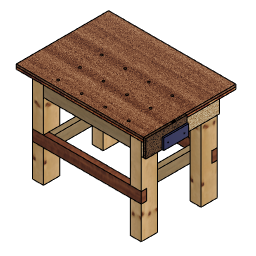
workbench (Autodesk Fusion 360 design; units mm, degrees)
Autodesk Fusion 360 part; units mm, degrees
note: some values were not read from the file. Set by a fixed rule: which face or edge a step refers to.
sketch "Sketch1" plane through (0, 0, 0) normal (0, 0, 1) x (1, 0, 0)
  line L0 (0, 0) -> (100, 0)
  line L1 (100, 0) -> (100, 150)
  line L2 (100, 150) -> (0, 150)
  line L3 (0, 150) -> (0, 0)
  dimension "d1" = 100
  dimension "d2" = 150
  constraint horizontal L0
  constraint vertical L1
  constraint horizontal L2
  constraint vertical L3
  constraint coincident L0.start L3.end
  measures "d1" distance of L0.start L0.end
  measures "d2" distance of L0.start L2.end
extrude "Extrude1" add sketch "Sketch1" along normal blind 800 makes body 1
sketch "Sketch2" plane through (0, 0, 0) normal (-1, 0, 0) x (0, -1, 0)
  line L0 (-150, 0) -> (0, 0)
  line L1 (0, 0) -> (0, 800)
  line L2 (0, 800) -> (-150, 800)
  line L3 (-150, 800) -> (-150, 0)
  line L4 (0, 300) -> (-50, 300)
  line L5 (-50, 300) -> (-50, 400)
  line L6 (-50, 400) -> (0, 400)
  line L7 (0, 400) -> (0, 300)
  dimension "d5" = 50
  dimension "d6" = 100
  constraint horizontal L4
  constraint vertical L5
  constraint horizontal L6
  constraint vertical L7
  constraint coincident L1 L4.start
  measures "d5" distance of L4.start L4.end
  measures "d6" distance of L4.end L5.end
extrude "Extrude2" cut sketch "Sketch2" against normal blind 100 contours L1 L4 L5 L6 L7 bodies 1
sketch "Sketch4" plane through (0, 150, 0) normal (0, -1, 0) x (1, 0, 0)
  line L0 (0, 400) -> (100, 400)
  line L1 (100, 400) -> (100, 800)
  line L2 (100, 800) -> (0, 800)
  line L3 (0, 800) -> (0, 400)
  line L4 (0, 800) -> (150, 800)
  line L5 (150, 800) -> (150, 700)
  line L6 (150, 700) -> (0, 700)
  line L7 (0, 700) -> (0, 800)
  line L8 (100, 0) -> (0, 0)
  line L9 (0, 0) -> (0, 800)
  line L10 (0, 800) -> (100, 800)
  line L11 (100, 800) -> (100, 0)
  dimension "d15" = 100
  dimension "d16" = 150
  constraint horizontal L4
  constraint vertical L5
  constraint horizontal L6
  constraint vertical L7
  constraint coincident L2.end L3.start
  measures "d15" distance of L2.end L6.end
  measures "d16" distance of L2.end L4.end
extrude "Extrude5" cut sketch "Sketch4" along normal blind 100 contours L1 L2 L3 L4 L6 L7 L9 L10 L11 | L1 L4 L5 L6 L11 bodies 1
extrude "Extrude6" add sketch "Sketch2" against normal blind 1000 separate body contours L1 L4 L5 L6 L7 makes body 2
extrude "Extrude7" add sketch "Sketch4" against normal blind 500 separate body contours L1 L2 L3 L4 L6 L7 L9 L10 L11 | L1 L4 L5 L6 L11 makes body 3
extrude "Extrude10" add 1 faces at (33.3333, 150, 766.6667) along direction (0, -1, 0) blind 100 on bodies 3 bodies 3
mirror "Mirror1" about plane through (0, 0, 0) normal (1, 0, 0) of bodies 1 makes body 4
move_body "Move3" bodies 4 to x (1, 0, 0) y (0, 1, 0) z (0, 0, 1) at (1000, 0, 0)
copy_body "CopyPasteBodies3" bodies 3 makes body 5
move_body "Move4" bodies 5 to x (1, 0, 0) y (0, 1, 0) z (0, 0, 1) at (850, 0, 0)
mirror "Mirror2" about plane through (0, 0, 0) normal (0, 1, 0) of bodies 1 makes body 6
move_body "Move5" bodies 6 to x (1, 0, 0) y (0, 1, 0) z (0, 0, 1) at (0, 700, 0)
copy_body "CopyPasteBodies4" bodies 2 makes body 7
move_body "Move6" bodies 7 to x (1, 0, 0) y (0, 1, 0) z (0, 0, 1) at (0, 650, 0)
mirror "Mirror3" about plane through (0, 0, 0) normal (1, 0, 0) of bodies 6 makes body 8
move_body "Move7" bodies 8 to x (1, 0, 0) y (0, 1, 0) z (0, 0, 1) at (1000, 0, 0)
sketch "Sketch5" plane through (0, 650, 0) normal (0, -1, 0) x (1, 0, 0)
  line L0 (0, 400) -> (0, 300)
  line L1 (0, 300) -> (1000, 300)
  line L2 (1000, 300) -> (1000, 400)
  line L3 (1000, 400) -> (0, 400)
  line L4 (100, 400) -> (150, 400)
  line L5 (150, 400) -> (150, 300)
  line L6 (150, 300) -> (100, 300)
  line L7 (100, 300) -> (100, 400)
  constraint horizontal L4
  constraint vertical L5
  constraint horizontal L6
  constraint vertical L7
  constraint coincident L1 L5.end
  constraint coincident L3 L4.start
extrude "Extrude8" add sketch "Sketch5" along normal blind 600 separate body contours L1 L3 L4 L5 L6 L7 makes body 9
copy_body "CopyPasteBodies5" bodies 9 makes body 10
move_body "Move8" bodies 10 to x (1, 0, 0) y (0, 1, 0) z (0, 0, 1) at (750, 0, 0)
sketch "Sketch7" plane through (100, 0, 0) normal (1, 0, 0) x (0, 1, 0)
  line L0 (50, 700) -> (50, 800)
  line L1 (50, 800) -> (0, 800)
  line L2 (0, 800) -> (0, 400)
  line L3 (0, 400) -> (50, 400)
  line L4 (50, 400) -> (50, 300)
  line L5 (50, 300) -> (0, 300)
  line L6 (0, 300) -> (0, 0)
  line L7 (0, 0) -> (150, 0)
  line L8 (150, 0) -> (150, 700)
  line L9 (150, 700) -> (50, 700)
  line L10 (0, 800) -> (50, 800)
  line L11 (50, 800) -> (50, 700)
  line L12 (50, 700) -> (0, 700)
  line L13 (0, 700) -> (0, 800)
  constraint horizontal L10
  constraint vertical L11
  constraint horizontal L12
  constraint vertical L13
  constraint coincident L0.start L9.end
  constraint coincident L1.end L2.start
extrude "Extrude11" add sketch "Sketch7" along normal blind 800 separate body contours L0 L1 L2 L10 L11 L12 L13 makes body 11
copy_body "CopyPasteBodies6" bodies 11 makes body 12
move_body "Move9" bodies 12 to x (1, 0, 0) y (0, 1, 0) z (0, 0, 1) at (0, 650, 0)
sketch "Sketch8" plane through (0, 0, 800) normal (0, 0, 1) x (-1, 0, 0)
  line L0 (-1000, -50) -> (-900, -50)
  line L1 (-900, -50) -> (-900, 0)
  line L2 (-900, 0) -> (-1000, 0)
  line L3 (-1000, 0) -> (-1000, -50)
  line L4 (-1000, 0) -> (150, 0)
  line L5 (150, 0) -> (150, -850)
  line L6 (150, -850) -> (-1000, -850)
  line L7 (-1000, -850) -> (-1000, 0)
  constraint horizontal L4
  constraint vertical L5
  constraint horizontal L6
  constraint vertical L7
  constraint coincident L2.end L3.start
extrude "Extrude12" add sketch "Sketch8" along normal blind 21 separate body makes body 13
copy_body "CopyPasteBodies7" bodies 13 makes body 14
move_body "Move10" bodies 14 to x (1, 0, 0) y (0, 1, 0) z (0, 0, 1) at (0, 0, 21)
sketch "Sketch9" plane through (1000, 0, 0) normal (1, 0, 0) x (0, 1, 0)
  line L0 (50, 700) -> (650, 700)
  line L1 (650, 700) -> (650, 800)
  line L2 (650, 800) -> (50, 800)
  line L3 (50, 800) -> (50, 700)
  line L4 (150, 700) -> (380, 700)
  line L5 (380, 700) -> (380, 780)
  line L6 (380, 780) -> (150, 780)
  line L7 (150, 780) -> (150, 700)
  dimension "d39" = 230
  dimension "d40" = 80
  constraint horizontal L4
  constraint vertical L5
  constraint horizontal L6
  constraint vertical L7
  constraint coincident L0 L4.start
  measures "d39" distance of L5.end L6.end
  measures "d40" distance of L4.start L6.end
extrude "Extrude14" cut sketch "Sketch9" against normal blind 15 contours L0 L4 L5 L6 L7 bodies 5
extrude "Extrude15" add 1 faces at (985, 226.6667, 753.3333) along direction (1, 0, 0) blind 15 separate body on bodies 5 makes body 15
extrude "Extrude16" add 1 faces at (990, 226.6667, 700) along direction (0, 0, -1) blind 20 on bodies 15 bodies 15
sketch "Sketch10" plane through (985, 0, 0) normal (-1, 0, 0) x (0, -1, 0)
  line L0 (-150, 680) -> (-150, 780)
  line L1 (-150, 780) -> (-380, 780)
  line L2 (-380, 780) -> (-380, 680)
  line L3 (-380, 680) -> (-150, 680)
  line L4 (-380, 680) -> (-150, 680)
  line L5 (-150, 680) -> (-150, 700)
  line L6 (-150, 700) -> (-380, 700)
  line L7 (-380, 700) -> (-380, 680)
  constraint horizontal L4
  constraint vertical L5
  constraint horizontal L6
  constraint vertical L7
  constraint coincident L0 L5.end
  constraint coincident L2.end L3.start
extrude "Extrude17" add sketch "Sketch10" along normal blind 120 contours L0 L2 L3 L4 L5 L6 L7 bodies 15
sketch "Sketch11" plane through (0, 0, 700) normal (0, 0, 1) x (-1, 0, 0)
  line L0 (-985, -150) -> (-985, -380)
  line L1 (-985, -380) -> (-865, -380)
  line L2 (-865, -380) -> (-865, -150)
  line L3 (-865, -150) -> (-985, -150)
  line L4 (-865, -150) -> (-985, -150)
  line L5 (-985, -150) -> (-985, -158.5)
  line L6 (-985, -158.5) -> (-865, -158.5)
  line L7 (-865, -158.5) -> (-865, -150)
  dimension "d49" = 8.5
  constraint horizontal L4
  constraint vertical L5
  constraint horizontal L6
  constraint vertical L7
  constraint coincident L0 L5.end
  constraint coincident L2.end L3.start
  measures "d49" distance of L2.end L6.end
extrude "Extrude18" cut sketch "Sketch11" against normal blind 20 contours L0 L2 L3 L4 L5 L6 L7 bodies 15
sketch "Sketch12" plane through (0, 0, 700) normal (0, 0, 1) x (-1, 0, 0)
  line L0 (-865, -158.5) -> (-985, -158.5)
  line L1 (-985, -158.5) -> (-985, -380)
  line L2 (-985, -380) -> (-865, -380)
  line L3 (-865, -380) -> (-865, -158.5)
  line L4 (-865, -380) -> (-985, -380)
  line L5 (-985, -380) -> (-985, -371.5)
  line L6 (-985, -371.5) -> (-865, -371.5)
  line L7 (-865, -371.5) -> (-865, -380)
  dimension "d52" = 8.5
  constraint horizontal L4
  constraint vertical L5
  constraint horizontal L6
  constraint vertical L7
  constraint coincident L1 L5.end
  constraint coincident L2.end L3.start
  measures "d52" distance of L2.end L6.end
extrude "Extrude19" cut sketch "Sketch12" against normal blind 20 contours L1 L2 L3 L4 L5 L6 L7 bodies 15
sketch "Sketch13" plane through (0, 0, 700) normal (0, 0, 1) x (-1, 0, 0)
  line L0 (-985, -371.5) -> (-865, -371.5)
  line L1 (-865, -371.5) -> (-865, -158.5)
  line L2 (-865, -158.5) -> (-985, -158.5)
  line L3 (-985, -158.5) -> (-985, -371.5)
  circle A0 centre (-962.5, -176) radius 7.5
  circle A1 centre (-962.5, -354) radius 7.5
  circle A2 centre (-885.5, -184) radius 7.5
  circle A3 centre (-885.5, -346) radius 7.5
  dimension "d55" = 15
  dimension "d56" = 17.5
  dimension "d57" = 22.5
  dimension "d58" = 15
  dimension "d59" = 17.5
  dimension "d60" = 22.5
  dimension "d61" = 15
  dimension "d62" = 15
  dimension "d63" = 99.5
  dimension "d64" = 99.5
  dimension "d65" = 25.5
  dimension "d66" = 25.5
  measures "d55" diameter of A0
  measures "d56" distance of L2 A0.centre
  measures "d57" distance of L3 A0.centre
  measures "d58" diameter of A1
  measures "d59" distance of L0 A1.centre
  measures "d60" distance of L3 A1.centre
  measures "d61" diameter of A2
  measures "d62" diameter of A3
  measures "d63" distance of L3 A2.centre
  measures "d64" distance of L3 A3.centre
  measures "d65" distance of L2 A2.centre
  measures "d66" distance of L0 A3.centre
extrude "Extrude20" cut sketch "Sketch13" against normal blind 20 contours A0 | A1 | A2 | A3 bodies 15
sketch "Sketch14" plane through (985, 0, 0) normal (-1, 0, 0) x (0, -1, 0)
  line L0 (-371.5, 700) -> (-158.5, 700)
  line L1 (-158.5, 700) -> (-158.5, 680)
  line L2 (-158.5, 680) -> (-150, 680)
  line L3 (-150, 680) -> (-150, 780)
  line L4 (-150, 780) -> (-380, 780)
  line L5 (-380, 780) -> (-380, 680)
  line L6 (-380, 680) -> (-371.5, 680)
  line L7 (-371.5, 680) -> (-371.5, 700)
  circle A0 centre (-340, 724) radius 4
  circle A1 centre (-190, 724) radius 4
  dimension "d69" = 8
  dimension "d70" = 8
  dimension "d71" = 40
  dimension "d72" = 40
  dimension "d73" = 56
  dimension "d74" = 56
  measures "d69" diameter of A0
  measures "d70" diameter of A1
  measures "d71" distance of L5 A0.centre
  measures "d72" distance of L3 A1.centre
  measures "d73" distance of L4 A0.centre
  measures "d74" distance of L4 A1.centre
extrude "Extrude21" cut sketch "Sketch14" against normal blind 15 contours A0 | A1 bodies 15
sketch "Sketch15" plane through (1000, 0, 0) normal (1, 0, 0) x (0, 1, 0)
  circle A0 centre (340, 724) radius 4
  circle A1 centre (190, 724) radius 4
  line L0 (150, 780) -> (150, 680)
  line L1 (150, 680) -> (380, 680)
  line L2 (380, 680) -> (380, 780)
  line L3 (380, 780) -> (150, 780)
  line L4 (380, 680) -> (0, 680)
  line L5 (0, 680) -> (0, 800)
  line L6 (0, 800) -> (380, 800)
  line L7 (380, 800) -> (380, 680)
  dimension "d77" = 380
  constraint horizontal L4
  constraint vertical L5
  constraint horizontal L6
  constraint vertical L7
  constraint coincident L1.end L2.start
  measures "d77" distance of L5.end L6.end
extrude "Extrude22" add sketch "Sketch15" along normal blind 21 separate body makes body 16
copy_body "CopyPasteBodies8" bodies 16 makes body 17
move_body "Move11" bodies 17 to x (1, 0, 0) y (0, 1, 0) z (0, 0, 1) at (21, 0, 0)
extrude "Extrude23" add 2 faces at (1007, 380, 713.3333) (1007, 380, 793.3333) along direction (0, 1, 0) blind 320 on bodies 16 bodies 16
extrude "Extrude24" add 2 faces at (1000, 16.6667, 807) (1000, 583.3333, 814) along direction (1, 0, 0) blind 21 on bodies 13 bodies 13
extrude "Extrude25" add 2 faces at (1000, 16.6667, 828) (1000, 583.3333, 835) along direction (1, 0, 0) blind 21 on bodies 14 bodies 14
extrude "Extrude26" add 1 faces at (1028, 126.6667, 800) along direction (0, 0, 1) blind 42 on bodies 17 bodies 17
sketch "Sketch17" plane through (0, 0, 842) normal (0, 0, 1) x (-1, 0, 0)
  line L0 (-1021, -850) -> (150, -850)
  line L1 (150, -850) -> (150, 0)
  line L2 (150, 0) -> (-1021, 0)
  line L3 (-1021, 0) -> (-1021, -850)
  circle A0 centre (-821, -265) radius 10
  circle A1 centre (-821, -65) radius 10
  circle A2 centre (-604.3333, -65) radius 10
  circle A3 centre (-604.3333, -265) radius 10
  circle A4 centre (-387.6667, -265) radius 10
  circle A5 centre (-387.6667, -65) radius 10
  circle A6 centre (-171, -65) radius 10
  circle A7 centre (-171, -265) radius 10
  line L4 (-821, -265) -> (-1058.3995, -265) construction
  line L5 (-1036.8104, -250) -> (-1026.8104, -250)
  line L6 (-1026.8104, -250) -> (-1026.8104, -280)
  line L7 (-1026.8104, -280) -> (-1036.8104, -280)
  line L8 (-1036.8104, -280) -> (-1036.8104, -250)
  line L9 (-1036.8104, -250) -> (-1026.8104, -280) construction
  line L10 (-1026.8104, -250) -> (-1036.8104, -280) construction
  line L11 (-985, -150) -> (-1000, -150)
  circle A8 centre (-821, -465) radius 10
  circle A9 centre (-604.3333, -465) radius 10
  circle A10 centre (-387.6667, -465) radius 10
  circle A11 centre (-171, -465) radius 10
  point P0 (-1031.8104, -265)
  dimension "d92" = 20
  dimension "d93" = 265
  dimension "d94" = 200
  dimension "d99" = 650
  dimension "d100" = -200
  dimension "d103" = 10
  dimension "d104" = 30
  dimension "d109" = 115
  constraint coincident A0.centre L4.start
  constraint horizontal L5
  constraint perpendicular L5 L6
  constraint parallel L5 L7
  constraint parallel L6 L8
  constraint coincident L9 P0
  constraint coincident L10 P0
  constraint coincident L4 P0
  constraint parallel L2 L4
  measures "d92" diameter of A0
  measures "d93" distance of L2 A0.centre
  measures "d94" distance of L3 A0.centre
  measures "d103" distance of L6.end L7.end
  measures "d104" distance of L5.end L6.end
  measures "d109" distance of P0 L11
extrude "Extrude28" cut sketch "Sketch17" against normal blind 42 contours A0 | A1 | A2 | A3 | A4 | A5 | A6 | A7 | L5 L6 L7 L8 | A8 | A9 | A10 | A11 bodies 17 14 13
sketch "Sketch16" plane through (1042, 0, 0) normal (1, 0, 0) x (0, 1, 0)
  circle A0 centre (190, 724) radius 4
  circle A1 centre (340, 724) radius 4
  line L0 (0, 842) -> (0, 680)
  line L1 (0, 680) -> (380, 680)
  line L2 (380, 680) -> (380, 842)
  line L3 (380, 842) -> (0, 842)
  line L4 (380, 680) -> (150, 680)
  line L5 (150, 680) -> (150, 780)
  line L6 (150, 780) -> (380, 780)
  line L7 (380, 780) -> (380, 680)
  dimension "d88" = 230
  dimension "d89" = 100
  constraint horizontal L4
  constraint vertical L5
  constraint horizontal L6
  constraint vertical L7
  constraint coincident L1.end L2.start
  measures "d88" distance of L5.end L6.end
  measures "d89" distance of L1.end L6.end
extrude "Extrude27" add sketch "Sketch16" along normal blind 15 separate body contours L1 L2 L4 L5 L6 L7 makes body 18
copy_body "Body->Comp1" bodies 1 removing the originals makes body 19 in component "ножка"
copy_body "Body->Comp2" bodies 2 removing the originals makes body 20 in component "перекладина длинная низ"
copy_body "Body->Comp3" bodies 7 removing the originals makes body 21 in component "перекладина длинная низ (1)"
copy_body "Body->Comp4" bodies 9 removing the originals makes body 22 in component "перекладина короткая низ"
copy_body "Body->Comp5" bodies 10 removing the originals makes body 23 in component "перекладина короткая низ (1)"
copy_body "Body->Comp6" bodies 3 removing the originals makes body 24 in component "перекладина короткая верх"
copy_body "Body->Comp7" bodies 4 removing the originals makes body 25 in component "ножка (1)"
copy_body "Body->Comp8" bodies 5 removing the originals makes body 26 in component "перекладина короткая верх (1)"
copy_body "Body->Comp9" bodies 6 removing the originals makes body 27 in component "ножка (2)"
copy_body "Body->Comp10" bodies 8 removing the originals makes body 28 in component "ножка (2) (1)"
copy_body "Body->Comp11" bodies 11 removing the originals makes body 29 in component "перекладина длинная верх"
copy_body "Body->Comp12" bodies 12 removing the originals makes body 30 in component "перекладина длинная верх (1)"
copy_body "Body->Comp13" bodies 13 removing the originals makes body 31 in component "столешница (фанера)"
copy_body "Body->Comp14" bodies 14 removing the originals makes body 32 in component "столешница (фанера)(1)"
copy_body "Body->Comp15" bodies 16 removing the originals makes body 33 in component "фанера"
copy_body "Body->Comp16" bodies 17 removing the originals makes body 34 in component "фанера (1)"
copy_body "Body->Comp17" bodies 15 removing the originals makes body 35 in component "тиски"
copy_body "Body->Comp18" bodies 18 removing the originals makes body 36 in component "тиски 2"
component "ножка" placed x (1, 0, 0) y (0, 1, 0) z (0, 0, 1) at (0, 0, 0)
component "перекладина длинная низ" placed x (1, 0, 0) y (0, 1, 0) z (0, 0, 1) at (0, 0, 0)
component "перекладина длинная низ (1)" placed x (1, 0, 0) y (0, 1, 0) z (0, 0, 1) at (0, 0, 0)
component "перекладина короткая низ" placed x (1, 0, 0) y (0, 1, 0) z (0, 0, 1) at (0, 0, 0)
component "перекладина короткая низ (1)" placed x (1, 0, 0) y (0, 1, 0) z (0, 0, 1) at (0, 0, 0)
component "перекладина короткая верх" placed x (1, 0, 0) y (0, 1, 0) z (0, 0, 1) at (0, 0, 0)
component "ножка (1)" placed x (1, 0, 0) y (0, 1, 0) z (0, 0, 1) at (0, 0, 0)
component "перекладина короткая верх (1)" placed x (1, 0, 0) y (0, 1, 0) z (0, 0, 1) at (0, 0, 0)
component "ножка (2)" placed x (1, 0, 0) y (0, 1, 0) z (0, 0, 1) at (0, 0, 0)
component "ножка (2) (1)" placed x (1, 0, 0) y (0, 1, 0) z (0, 0, 1) at (0, 0, 0)
component "перекладина длинная верх" placed x (1, 0, 0) y (0, 1, 0) z (0, 0, 1) at (0, 0, 0)
component "перекладина длинная верх (1)" placed x (1, 0, 0) y (0, 1, 0) z (0, 0, 1) at (0, 0, 0)
component "столешница (фанера)" placed x (1, 0, 0) y (0, 1, 0) z (0, 0, 1) at (0, 0, 0)
component "столешница (фанера)(1)" placed x (1, 0, 0) y (0, 1, 0) z (0, 0, 1) at (0, 0, 0)
component "фанера" placed x (1, 0, 0) y (0, 1, 0) z (0, 0, 1) at (0, 0, 0)
component "фанера (1)" placed x (1, 0, 0) y (0, 1, 0) z (0, 0, 1) at (0, 0, 0)
component "тиски" placed x (1, 0, 0) y (0, 1, 0) z (0, 0, 1) at (0, 0, 0)
component "тиски 2" placed x (1, 0, 0) y (0, 1, 0) z (0, 0, 1) at (0, 0, 0)
equation "d56 = 10 mm + ( 15 / 2 ) * 1 mm"
equation "d57 = 15 mm + ( 15 / 2 ) * 1 mm"
equation "d59 = 10 mm + ( 15 / 2 ) * 1 mm"
equation "d60 = 15 mm + ( 15 / 2 ) * 1 mm"
equation "d63 = 92 mm + ( 15 / 2 ) * 1 mm"
equation "d64 = 92 mm + ( 15 / 2 ) * 1 mm"
equation "d65 = 18 mm + ( 15 / 2 ) * 1 mm"
equation "d66 = 18 mm + ( 15 / 2 ) * 1 mm"
equation "d71 = 36 mm + 4 mm"
equation "d72 = 36 mm + 4 mm"
equation "d73 = 52 mm + 4 mm"
equation "d74 = 52 mm + 4 mm"
named bodies: "ножка", "перекладина длинная низ", "перекладина короткая верх", "ножка (1)", "перекладина короткая верх (1)", "ножка (2)", "перекладина длинная низ (1)", "ножка (2) (1)", "перекладина короткая низ", "перекладина короткая низ (1)", "перекладина длинная верх", "перекладина длинная верх (1)", "столешница (фанера)", "столешница", "столешница (фанера)(1)", "тиски", "фанера", "фанера (1)", "тиски 2"
